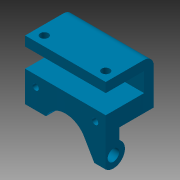
# Autodesk Inventor part: Part1
Saved by Autodesk Inventor 2015 (Build 190159000, 159)
## iProperties
Created: 2015-07-07
Part Number: Part1
Material: ABS Plastic
Document SubType Name: Modeling
Designer: eefred
Density: 1.06 g/cm^3
Appearance: Sky Blue Medium
Author: eefred
Autodesk Inventor part; units mm, degrees
ref_plane "YZ Plane" through (0, 0, 0) normal (1, 0, 0) x (0, 1, 0)
ref_plane "XZ Plane" through (0, 0, 0) normal (0, 1, 0) x (-1, 0, 0)
ref_plane "XY Plane" through (0, 0, 0) normal (0, 0, 1) x (1, 0, 0)
sketch "Sketch1" plane through (0, 0, 0) normal (1, 0, 0) x (0, 1, 0)
  line L0 (0, 0) -> (0, -5)
  line L1 (0, -5) -> (20, -5)
  line L2 (20, -5) -> (20, -15)
  line L3 (20, -15) -> (0, -15)
  line L4 (0, -15) -> (0, -39.4721)
  line L5 (25, 0) -> (25, -24)
  line L6 (25, -24) -> (7, -24)
  line L7 (7, -24) -> (7, -29.8038)
  line L8 (25, 0) -> (0, 0)
  circle A0 centre (4, -35) radius 3
  arc A1 (0, -39.4721) -> (7, -29.8038) centre (4, -35) ccw
  dimension "d0" = 5
  dimension "d1" = 20
  dimension "d2" = 10
  dimension "d5" = 5
  dimension "d6" = 7
  dimension "d7" = 6
  dimension "d8" = 20
  dimension "d9" = 4
  dimension "d10" = 6
  dimension "d45" = 9
  constraints: 18 end point, 3 perpendicular, 2 centre point, 2 horizontal, 2 point on circle, 2 point on line, 2 vertical, 1 coincident, 1 parallel
  measures "d0" distance of L0.start L0.end
  measures "d1" distance of L0.end L1.end
  measures "d2" distance of L1.end L2.end
  measures "d5" distance between parallel lines of L5 L2
  measures "d6" distance between parallel lines of L4 L7
  measures "d7" diameter of A0
  measures "d8" distance from line of L3 A0.centre
  measures "d9" distance from line of L4 A0.centre
  measures "d10" radius of A1
  measures "d45" distance between parallel lines of L6 L3
extrude "Extrusion1" add sketch "Sketch1" along normal blind 42
fillet "Fillet1" radius 5 1 edges at (21, 25, 0)
sketch "Sketch2" plane through (0, 7, -24) normal (0, 1, 0) x (1, 0, 0)
  arc A0 (10.8664, 7) -> (31.1336, 7) centre (21, 12) ccw
  line L0 (0, 0) -> (42, 0) projected
  line L1 (10.8664, 7) -> (3.3664, 19.9904)
  line L2 (10.8664, 7) -> (25.8664, 7) construction
  line L3 (31.1336, 7) -> (38.6336, 19.9904)
  line L4 (31.1336, 7) -> (46.1336, 7) construction
  line L5 (38.6336, 19.9904) -> (3.3664, 19.9904)
  line L6 (0, 0) -> (42, 0) projected
  point P0 (0, -24)
  point P1 (21, 0)
  dimension "d14" = 11.3
  dimension "d15" = 12
  dimension "d16" = 7
  dimension "d17" = 15
  dimension "d18" = 120
  dimension "d19" = 15
  dimension "d20" = 60
  constraints: 10 end point, 2 equal length, 2 horizontal, 2 point on circle, 1 centre point, 1 horizontal alignment, 1 midpoint, 1 vertical alignment
  measures "d14" radius of A0
  measures "d15" distance from line of A0.centre L0
  measures "d16" distance from line of L0 L1.start
  measures "d17" distance of L1.start L1.end
  measures "d18" angle of L2 L1
  measures "d19" distance of L3.start L3.end
  measures "d20" angle of L4 L3
extrude "Extrusion2" cut sketch "Sketch2" along normal through all both and the other way through all
sketch "Sketch3" plane through (42, 0, 0) normal (1, 0, 0) x (0, 0, -1)
  line L0 (29, 7) -> (31, 7)
  line L1 (31, 7) -> (31, 0)
  line L2 (31, 0) -> (43, 0)
  line L3 (43, 0) -> (43, 12)
  line L4 (43, 12) -> (29, 12)
  line L5 (29, 12) -> (29, 7)
  line L6 (15, 20) -> (15, 0) projected
  point P0 (0, 0)
  dimension "d23" = 7
  dimension "d24" = 16
  dimension "d25" = 2
  dimension "d26" = 12
  dimension "d27" = 14
  constraints: 12 end point, 5 perpendicular, 1 horizontal, 1 horizontal alignment
  measures "d23" distance between parallel lines of L2 L0
  measures "d24" distance between parallel lines of L6 L1
  measures "d25" distance of L0.start L0.end
  measures "d26" distance of L2.end L3.end
  measures "d27" distance of L3.end L4.end
extrude "Extrusion3" cut sketch "Sketch3" against normal up to surface round surface about axis through (21, 7, -36) along (0, 1, 0) radius 11.3 far side no
sketch "Sketch4" plane through (0, 25, -24) normal (0, 1, 0) x (1, 0, 0)
  circle A0 centre (5.5, -3.5) radius 1.6
  circle A1 centre (36.5, -3.5) radius 1.6
  line L0 (0, 0) -> (0, -19) projected
  line L1 (42, 0) -> (42, -19) projected
  line L2 (0, 0) -> (42, 0) projected
  point P0 (0, -24)
  dimension "d30" = 3.2
  dimension "d31" = 5.5
  dimension "d32" = 5.5
  dimension "d33" = 3.5
  dimension "d34" = 3.5
  constraints: 2 centre point, 1 equal radius
  measures "d30" diameter of A0
  measures "d31" distance from line of L0 A0.centre
  measures "d32" distance from line of L1 A1.centre
  measures "d33" distance from line of A1.centre L2
  measures "d34" distance from line of A0.centre L2
extrude "Extrusion4" cut sketch "Sketch4" against normal through all
sketch "Sketch5" plane through (0, 0, 0) normal (0, 0, 1) x (1, 0, 0)
  circle A0 centre (5, 5) radius 2.1
  circle A1 centre (37, 5) radius 2.1
  line L0 (0, 0) -> (42, 0) projected
  line L1 (0, 20) -> (0, 0) projected
  line L2 (42, 20) -> (42, 0) projected
  dimension "d37" = 4.2
  dimension "d38" = 5
  dimension "d39" = 5
  dimension "d40" = 5
  constraints: 2 centre point, 1 equal radius, 1 horizontal alignment
  measures "d37" diameter of A0
  measures "d38" distance from line of A0.centre L0
  measures "d39" distance from line of L1 A0.centre
  measures "d40" distance from line of L2 A1.centre
extrude "Extrusion5" cut sketch "Sketch5" against normal up to next
mirror "Mirror1" about plane through (0, 0, 0) normal (1, 0, 0) remove original yes
sketch "Sketch6" plane through (0, 25, -5) normal (0, 1, 0) x (1, 0, 0)
  line L0 (-18.3728, 14.8357) -> (-18.2457, 14.9083)
  spline S0 degree 2 poles (-18.2457, 14.9083) (-17.9915, 15.0718) (-17.8643, 15.0718) knots 0 0 0 1 1 1
  spline S1 degree 2 poles (-17.8643, 15.0718) (-17.6101, 15.0718) (-17.2468, 14.5633) (-17.2468, 14.3544) knots 0 0 0 1 2 2 2
  spline S2 degree 2 poles (-17.2468, 14.3544) (-17.2468, 14.2636) (-17.2559, 14.1183) knots 0 0 0 1 1 1
  spline S3 degree 2 poles (-17.2559, 14.1183) (-17.2832, 13.973) (-17.2832, 13.9367) knots 0 0 0 1 1 1
  spline S4 degree 2 poles (-17.2832, 13.9367) (-17.038, 12.4021) (-17.038, 11.7846) knots 0 0 0 1 1 1
  spline S5 degree 2 poles (-17.038, 11.7846) (-17.038, 10.6223) (-18.1367, 9.2693) (-18.9449, 9.2693) knots 0 0 0 1 2 2 2
  spline S6 degree 2 poles (-18.9449, 9.2693) (-19.7168, 9.2693) (-21.1061, 10.5951) (-21.551, 11.712) knots 0 0 0 1 2 2 2
  spline S7 degree 2 poles (-21.551, 11.712) (-23.0493, 9.8595) (-23.6123, 8.897) knots 0 0 0 1 1 1
  spline S8 degree 2 poles (-23.6123, 8.897) (-23.8121, 8.561) (-24.1299, 8.561) knots 0 0 0 1 1 1
  spline S9 degree 2 poles (-24.1299, 8.561) (-24.3388, 8.561) (-24.7565, 9.0332) (-24.7565, 9.242) knots 0 0 0 1 2 2 2
  spline S10 degree 2 poles (-24.7565, 9.242) (-24.7565, 9.5508) (-24.2389, 10.3136) (-23.1129, 11.721) (-23.0039, 11.83) knots 0 0 0 1 2 3 3 3
  spline S11 degree 2 poles (-23.0039, 11.83) (-22.1776, 12.8198) (-21.9052, 13.2647) knots 0 0 0 1 1 1
  spline S12 degree 2 poles (-21.9052, 13.2647) (-21.9052, 13.8096) (-21.3604, 13.8096) knots 0 0 0 1 1 1
  spline S13 degree 2 poles (-21.3604, 13.8096) (-21.1061, 13.8096) (-20.7338, 13.3283) (-20.7338, 13.0105) knots 0 0 0 1 2 2 2
  spline S14 degree 2 poles (-20.7338, 13.0105) (-20.7338, 12.9197) (-20.761, 12.8198) knots 0 0 0 1 1 1
  spline S15 degree 2 poles (-20.761, 12.8198) (-20.7883, 12.7199) (-20.7883, 12.6745) knots 0 0 0 1 1 1
  spline S16 degree 2 poles (-20.7883, 12.6745) (-20.7883, 12.3476) (-19.6804, 10.5406) (-18.9449, 10.5406) knots 0 0 0 1 2 2 2
  spline S17 degree 2 poles (-18.9449, 10.5406) (-18.5817, 10.5406) (-18.0641, 11.2943) (-18.0641, 11.8845) knots 0 0 0 1 2 2 2
  spline S18 degree 2 poles (-18.0641, 11.8845) (-18.0641, 12.5746) (-18.2275, 13.4191) (-18.3002, 13.5008) (-18.5544, 13.6098) (-20.4341, 13.964) (-22.6861, 14.2545) (-23.2128, 14.2545) knots 0 0 0 1 2 3 4 5 6 6 6
  spline S19 degree 2 poles (-23.2128, 14.2545) (-23.5579, 14.2545) (-23.8212, 14.2) knots 0 0 0 1 1 1
  spline S20 degree 2 poles (-23.8212, 14.2) (-24.0936, 14.1546) (-24.2934, 14.1546) knots 0 0 0 1 1 1
  spline S21 degree 2 poles (-24.2934, 14.1546) (-24.4841, 14.1546) (-24.9109, 14.5996) (-24.9109, 14.8538) knots 0 0 0 1 2 2 2
  spline S22 degree 2 poles (-24.9109, 14.8538) (-24.9109, 15.5803) (-23.912, 15.5803) knots 0 0 0 1 1 1
  spline S23 degree 2 poles (-23.912, 15.5803) (-23.1038, 15.5803) (-20.1708, 15.2171) (-19.063, 14.9719) knots 0 0 0 1 2 2 2
  spline S24 degree 2 poles (-19.063, 14.9719) (-18.8814, 14.9356) (-18.7451, 14.9174) knots 0 0 0 1 1 1
  line L1 (-18.7451, 14.9174) -> (-18.3728, 14.8357)
  point P0 (0, -5)
  point P1 (-17.038, 16.2886)
  constraints: 1 other
extrude "Extrusion6" add sketch "Sketch6" along normal blind 0.6
equation "\"d32\" = d31"
equation "\"d40\" = d39"
body "Solid1"
